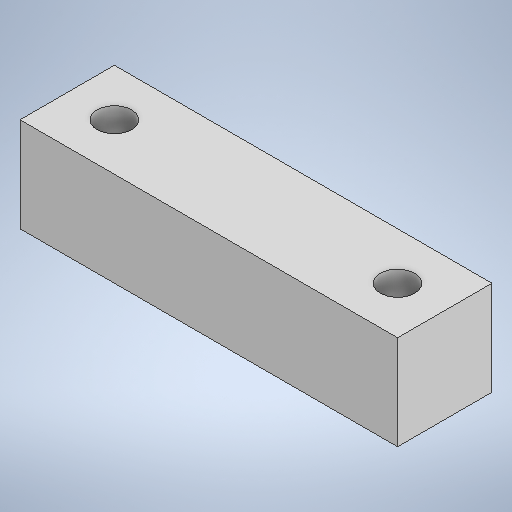
# Autodesk Inventor part: hinge align mech
Saved by Autodesk Inventor 2025.1 (Build 291241020, 241B)
## iProperties
Created: 2025-01-14
Part Number: hinge align mech
Material: Generic
Document SubType Name: Modeling
Designer: Hunter Mathis
Density: 1 g/cm^3
Appearance: Default
Author: Hunter Mathis
Autodesk Inventor part; units mm, degrees
ref_plane "YZ Plane" through (0, 0, 0) normal (1, 0, 0) x (0, 1, 0)
ref_plane "XZ Plane" through (0, 0, 0) normal (0, 1, 0) x (-1, 0, 0)
ref_plane "XY Plane" through (0, 0, 0) normal (0, 0, 1) x (1, 0, 0)
sketch "Sketch1" plane through (0, 0, 0) normal (0, 0, 1) x (1, 0, 0)
  line L0 (-25.4, 6.35) -> (25.4, 6.35)
  line L1 (25.4, 6.35) -> (25.4, -6.35)
  line L2 (25.4, -6.35) -> (-25.4, -6.35)
  line L3 (-25.4, -6.35) -> (-25.4, 6.35)
  line L4 (-25.4, 6.35) -> (25.4, -6.35) construction
  line L5 (25.4, 6.35) -> (-25.4, -6.35) construction
  point P0 (0, 0)
  dimension "d0" = 50.8
  dimension "d1" = 12.7
  constraints: 12 end point, 2 midpoint, 2 parallel, 1 horizontal, 1 perpendicular
  measures "d0" distance of L1.end L2.end
  measures "d1" distance of L0.end L1.end
extrude "Extrusion1" add sketch "Sketch1" along normal blind 12.7
sketch "Sketch3" plane through (-25.4, 6.35, 0) normal (0, 1, 0) x (1, 0, 0)
  line L0 (0, 0) -> (50.8, 0) projected
  line L1 (50.8, 0) -> (50.8, -6.35)
  line L2 (50.8, 0) -> (50.8, -12.7) projected
  line L3 (50.8, -6.35) -> (44.45, -6.35)
  circle A0 centre (44.45, -6.35) radius 2.3241
  circle A1 centre (31.75, -6.35) radius 2.3241
  circle A2 centre (19.05, -6.35) radius 2.3241
  circle A3 centre (6.35, -6.35) radius 2.3241
  point P0 (25.4, 0)
  dimension "d16" = 6.35
  dimension "d17" = 6.35
  dimension "d18" = 4.6482
  dimension "d21" = 12.7
  constraints: 4 centre point, 4 end point, 2 horizontal, 1 coincident, 1 midpoint, 6 other
  measures "d16" distance of L0.end L1.end
  measures "d17" distance of L1.end L3.end
  measures "d18" diameter of A0
  measures "d21" distance of A0.centre A1.centre
extrude "Extrusion3" cut sketch "Sketch3" against normal blind 12.7 contours A0 | A3
body "Solid1"
